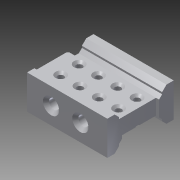
# Autodesk Inventor part: OnxyBelly
Saved by Autodesk Inventor 2015 (Build 190159000, 159)
## iProperties
Created: 2015-05-12
Part Number: OnxyBelly
Material: ABS Plastic
Document SubType Name: Modeling
Designer: Quinn
Density: 1.06 g/cm^3
Appearance: Smooth - White
Author: Quinn
Autodesk Inventor part; units mm, degrees
ref_plane "YZ Plane" through (0, 0, 0) normal (1, 0, 0) x (0, 1, 0)
ref_plane "XZ Plane" through (0, 0, 0) normal (0, 1, 0) x (-1, 0, 0)
ref_plane "XY Plane" through (0, 0, 0) normal (0, 0, 1) x (1, 0, 0)
sketch "Sketch1" plane through (0, 0, 0) normal (0, 1, 0) x (-1, 0, 0)
  line L0 (25, 21.5) -> (-25, 21.5)
  line L1 (-25, 21.5) -> (-25, -21.5)
  line L2 (-25, -21.5) -> (25, -21.5)
  line L3 (25, -21.5) -> (25, 21.5)
  line L4 (25, 21.5) -> (-25, 21.5)
  line L5 (-25, 21.5) -> (-25, 14)
  line L6 (-25, 14) -> (25, 14)
  line L7 (25, 14) -> (25, 21.5)
  line L8 (25, 0) -> (-25, 0)
  line L9 (-25, -14) -> (25, -14)
  line L10 (25, -14) -> (-25, -14)
  line L11 (-25, -14) -> (-25, -21.5)
  line L12 (-25, -21.5) -> (25, -21.5)
  line L13 (25, -21.5) -> (25, -14)
  point P0 (0, 0)
  point P1 (0, -21.5)
  dimension "d0" = 50
  dimension "d1" = 43
  dimension "d2" = 7.5
  constraints: 28 end point, 6 parallel, 3 horizontal, 3 midpoint, 3 perpendicular, 2 symmetric about line, 1 horizontal alignment, 1 point on line, 1 vertical alignment
  measures "d0" distance of L2.end L1.end
  measures "d1" distance of L1.end L0.end
  measures "d2" distance of L5.end L4.end
extrude "Extrusion1" add sketch "Sketch1" along normal blind 22 contours L3 L6 L1 L0 | L3 L2 L1 L9
ref_plane "Work Plane1" through (0, 11, 0) normal (0, 1, 0) x (1, 0, 0)
sketch "Sketch2" plane through (0, 11, 0) normal (0, 1, 0) x (1, 0, 0)
  line L0 (25, -14) -> (-25, -14) projected
  line L1 (25, -14) -> (-25, -14) projected
  line L2 (-25, 14) -> (25, 14) projected
  line L3 (-25, 14) -> (25, 14) projected
  line L4 (-25, -14) -> (25, -14)
  line L5 (25, -14) -> (25, 14)
  line L6 (25, 14) -> (-25, 14)
  line L7 (-25, 14) -> (-25, -14)
  point P0 (0, 0)
  constraints: 8 end point, 2 parallel, 1 horizontal, 1 perpendicular
extrude "Extrusion2" add sketch "Sketch2" along normal mid plane 10
chamfer "Chamfer1" distance 2 angle 45 4 edges at (0, 16, 14) (0, 16, -14) (0, 6, -14) (0, 6, 14)
sketch "Sketch3" plane through (0, 16, 0) normal (0, 1, 0) x (1, 0, 0)
  line L0 (-25, 12) -> (25, 12) projected
  line L1 (-25, 12) -> (-25, -12) projected
  line L2 (25, -12) -> (-25, -12) projected
  line L3 (25, -12) -> (25, 12) projected
  point P0 (0, 0)
sketch "Sketch4" plane through (0, 16, 0) normal (0, 1, 0) x (1, 0, 0)
  line L0 (25, 12) -> (-25, 12) projected
  line L1 (-25, 12) -> (25, 12) projected
  line L2 (-25, 12) -> (-25, -12) projected
  line L3 (25, -12) -> (-25, -12) projected
  line L4 (25, -12) -> (25, 12) projected
  line L5 (-25, 0) -> (25, 0)
  line L6 (-25, 0) -> (-25, -12)
  line L7 (-25, -6) -> (25, -6)
  line L8 (0, 0) -> (0, -12)
  line L9 (-25, 0) -> (-12.5, 0)
  line L10 (-12.5, 0) -> (-12.5, -12)
  line L11 (-18.75, 0) -> (-18.75, -12)
  circle A0 centre (-18.75, -6) radius 2
  circle A1 centre (-6.25, -6) radius 2
  circle A2 centre (6.25, -6) radius 2
  circle A3 centre (18.75, -6) radius 2
  circle A4 centre (-18.75, 6) radius 2
  circle A5 centre (-6.25, 6) radius 2
  circle A6 centre (6.25, 6) radius 2
  circle A7 centre (18.75, 6) radius 2
  dimension "d10" = 12.5
  dimension "d11" = 4
  dimension "d14" = 12.5
  constraints: 14 end point, 8 centre point, 6 midpoint, 4 point on line, 4 symmetric about line, 3 perpendicular, 1 collinear, 1 horizontal, 10 other
  measures "d10" distance of L5.start L9.end
  measures "d11" diameter of A0
  measures "d14" distance of A0.centre A1.centre
extrude "Extrusion3" cut sketch "Sketch4" against normal blind 27.4625 contours A3 L7 | L7 A3 | A0 L11 L7 | L7 L11 A0 | A0 L7 L11 | A1 L7 | L7 A1 | A2 L7 | L7 A2 | L7 A0 L11 | A4 | A5 | A6 | A7
chamfer "Chamfer2" distance 2.8 angle 45 4 edges at (0, 22, 14) (0, 22, -14) (0, 0, -14) (0, 0, 14)
sketch "Sketch5" plane through (-25, 0, 21.5) normal (-1, 0, 0) x (0, 0, 1)
  line L0 (-4.7, 0) -> (-7.5, 2.8) projected
  line L1 (-4.7, 0) -> (0, 0) projected
  line L2 (0, 0) -> (0, 22) projected
  line L3 (-4.7, 22) -> (0, 22) projected
  line L4 (-7.5, 19.2) -> (-4.7, 22) projected
  line L5 (-7.5, 18) -> (-7.5, 19.2) projected
  line L6 (-9.5, 16) -> (-7.5, 18) projected
  line L7 (-33.5, 16) -> (-9.5, 16) projected
  line L8 (-35.5, 18) -> (-33.5, 16) projected
  line L9 (-35.5, 18) -> (-35.5, 19.2) projected
  line L10 (-38.3, 22) -> (-35.5, 19.2) projected
  line L11 (-43, 22) -> (-38.3, 22) projected
  line L12 (-43, 0) -> (-43, 22) projected
  line L13 (-43, 0) -> (-38.3, 0) projected
  line L14 (-35.5, 2.8) -> (-38.3, 0) projected
  line L15 (-35.5, 2.8) -> (-35.5, 4) projected
  line L16 (-33.5, 6) -> (-35.5, 4) projected
  line L17 (-9.5, 6) -> (-33.5, 6) projected
  line L18 (-7.5, 4) -> (-9.5, 6) projected
  line L19 (-7.5, 2.8) -> (-7.5, 4) projected
  line L20 (-5.5, 3.6284) -> (-3.8716, 2)
  line L21 (-3.8716, 2) -> (-2, 2)
  line L22 (-2, 2) -> (-2, 20)
  line L23 (-2, 20) -> (-3.8716, 20)
  line L24 (-3.8716, 20) -> (-5.5, 18.3716)
  line L25 (-5.5, 18.3716) -> (-5.5, 17.1716)
  line L26 (-5.5, 17.1716) -> (-8.6716, 14)
  line L27 (-8.6716, 14) -> (-34.3284, 14)
  line L28 (-34.3284, 14) -> (-37.5, 17.1716)
  line L29 (-37.5, 17.1716) -> (-37.5, 18.3716)
  line L30 (-37.5, 18.3716) -> (-39.1284, 20)
  line L31 (-39.1284, 20) -> (-41, 20)
  line L32 (-41, 20) -> (-41, 2)
  line L33 (-41, 2) -> (-39.1284, 2)
  line L34 (-39.1284, 2) -> (-37.5, 3.6284)
  line L35 (-37.5, 3.6284) -> (-37.5, 4.8284)
  line L36 (-37.5, 4.8284) -> (-34.3284, 8)
  line L37 (-34.3284, 8) -> (-8.6716, 8)
  line L38 (-8.6716, 8) -> (-5.5, 4.8284)
  line L39 (-5.5, 4.8284) -> (-5.5, 3.6284)
  point P0 (-21.5, 0)
  dimension "d24" = 2
  constraints: 40 end point, 19 other
  measures "d24" distance between parallel lines of L0 L20
extrude "Extrusion4" cut sketch "Sketch5" against normal blind 2.5 contours L39 L38 L37 L36 L35 L34 L33 L32 L31 L30 L29 L28 L27 L26 L25 L24 L23 L22 L21 L20
sketch "Sketch6" plane through (-25, 0, 21.5) normal (0, 0, 1) x (1, 0, 0)
  line L0 (50, 16) -> (0, 16) projected
  line L1 (0, 6) -> (50, 6) projected
  line L2 (0, 0) -> (50, 0) projected
  line L3 (50, 0) -> (50, 22) projected
  line L4 (0, 22) -> (50, 22) projected
  line L5 (0, 0) -> (0, 22) projected
  line L6 (25, 0) -> (25, 22)
  line L7 (25, 11) -> (34.5, 11)
  line L8 (34.5, 11) -> (15.5, 11)
  circle A0 centre (34.5, 11) radius 3.25
  circle A1 centre (15.5, 11) radius 3.25
  dimension "d27" = 9.5
  dimension "d28" = 19
  dimension "d29" = 6.5
  dimension "d30" = 6.5
  constraints: 6 end point, 2 centre point, 2 coincident, 2 midpoint, 1 horizontal, 1 point on line
  measures "d27" distance of L7.start L7.end
  measures "d28" distance of L7.end L8.end
  measures "d29" diameter of A0
  measures "d30" diameter of A1
extrude "Extrusion5" cut sketch "Sketch6" against normal blind 6.5875 contours A0 | A1
mirror "Mirror1" about plane through (0, 0, 0) normal (0, 0, 1) of "Extrusion5"
chamfer "Chamfer3" distance 2 angle 45 4 edges at (-12.75, 11, -21.5) (6.25, 11, -21.5) (6.25, 11, 21.5) (-12.75, 11, 21.5)
chamfer "Chamfer4" distance 1.4 angle 45 16 edges at (-20.75, 6, 6) (-8.25, 6, 6) (4.25, 6, 6) (16.75, 6, 6) (16.75, 6, -6) (4.25, 6, -6) (-8.25, 6, -6) (-20.75, 6, -6) (-20.75, 16, -6) (-20.75, 16, 6) (-8.25, 16, 6) (-8.25, 16, -6) (4.25, 16, -6) (4.25, 16, 6) (16.75, 16, 6) (16.75, 16, -6)
sketch "Sketch7" plane through (25, 0, -21.5) normal (1, 0, 0) x (0, 0, -1)
  line L0 (-35.5, 2.8) -> (-38.3, 0) projected
  line L1 (-35.5, 2.8) -> (-35.5, 4) projected
  line L2 (-33.5, 6) -> (-35.5, 4) projected
  line L3 (-9.5, 6) -> (-33.5, 6) projected
  line L4 (-7.5, 4) -> (-9.5, 6) projected
  line L5 (-7.5, 2.8) -> (-7.5, 4) projected
  line L6 (-4.7, 0) -> (-7.5, 2.8) projected
  line L7 (-4.7, 0) -> (0, 0) projected
  line L8 (0, 0) -> (0, 22) projected
  line L9 (-4.7, 22) -> (0, 22) projected
  line L10 (-7.5, 19.2) -> (-4.7, 22) projected
  line L11 (-7.5, 18) -> (-7.5, 19.2) projected
  line L12 (-9.5, 16) -> (-7.5, 18) projected
  line L13 (-33.5, 16) -> (-9.5, 16) projected
  line L14 (-35.5, 18) -> (-33.5, 16) projected
  line L15 (-35.5, 18) -> (-35.5, 19.2) projected
  line L16 (-38.3, 22) -> (-35.5, 19.2) projected
  line L17 (-43, 22) -> (-38.3, 22) projected
  line L18 (-43, 0) -> (-43, 22) projected
  line L19 (-43, 0) -> (-38.3, 0) projected
  line L20 (-9.5, 6) -> (-33.5, 6)
  line L21 (-33.5, 6) -> (-33.5, 16)
  line L22 (-33.5, 16) -> (-9.5, 16)
  line L23 (-9.5, 16) -> (-9.5, 6)
  point P0 (-21.5, 0)
  constraints: 8 end point, 2 parallel, 1 horizontal, 1 perpendicular
extrude "Extrusion6" add sketch "Sketch7" along normal blind 2 contours L0 L19 L18 L17 L16 L15 L14 L21 L2 L1 | L23 L12 L11 L10 L9 L8 L7 L6 L5 L4
sketch "Sketch8" plane through (-22.5, 0, 21.5) normal (-1, 0, 0) x (0, 0, 1)
  line L0 (-3.8716, 2) -> (-5.5, 3.6284) projected
  line L1 (-2, 2) -> (-3.8716, 2) projected
  line L2 (-2, 20) -> (-2, 2) projected
  line L3 (-3.8716, 20) -> (-2, 20) projected
  line L4 (-5.5, 18.3716) -> (-3.8716, 20) projected
  line L5 (-5.5, 17.1716) -> (-5.5, 18.3716) projected
  line L6 (-8.6716, 14) -> (-5.5, 17.1716) projected
  line L7 (-34.3284, 14) -> (-8.6716, 14) projected
  line L8 (-37.5, 17.1716) -> (-34.3284, 14) projected
  line L9 (-37.5, 18.3716) -> (-37.5, 17.1716) projected
  line L10 (-39.1284, 20) -> (-37.5, 18.3716) projected
  line L11 (-41, 20) -> (-39.1284, 20) projected
  line L12 (-41, 2) -> (-41, 20) projected
  line L13 (-39.1284, 2) -> (-41, 2) projected
  line L14 (-37.5, 3.6284) -> (-39.1284, 2) projected
  line L15 (-37.5, 4.8284) -> (-37.5, 3.6284) projected
  line L16 (-34.3284, 8) -> (-37.5, 4.8284) projected
  line L17 (-8.6716, 8) -> (-34.3284, 8) projected
  line L18 (-5.5, 4.8284) -> (-8.6716, 8) projected
  line L19 (-5.5, 3.6284) -> (-5.5, 4.8284) projected
  line L20 (-8.6716, 8) -> (-8.6716, 14)
  line L21 (-2, 11) -> (-8.6716, 11)
  line L22 (-34.3284, 8) -> (-34.3284, 14)
  point P0 (-21.5, 0)
  constraints: 6 end point, 2 midpoint, 1 point on line, 1 vertical
ref_plane "Work Plane2" through (0, 11, 0) normal (0, -1, 0) x (1, 0, 0)
extrude "Extrusion7" add sketch "Sketch8" along normal blind 10 contours L17 L22 L7 L20
chamfer "Chamfer5" distance 1.4 angle 45 4 edges at (-28.75, 14, 12.8284) (-28.75, 14, -12.8284) (-28.75, 8, -12.8284) (-28.75, 8, 12.8284)
sketch "Sketch11" plane through (-32.5, 8, 11.4284) normal (0, -1, 0) x (1, 0, 0)
  line L0 (0, 0) -> (7.5, 0) projected
  line L1 (0, -22.8569) -> (0, 0) projected
  line L2 (7.5, -22.8569) -> (0, -22.8569) projected
  line L3 (7.5, 0) -> (7.5, -22.8569) projected
  line L4 (0, -22.8569) -> (3, -22.8569)
  line L5 (3, -22.8569) -> (3, 0)
  line L6 (3, 0) -> (0, 0)
  line L7 (0, 0) -> (0, -22.8569)
  line L8 (3, -11.4284) -> (0, -11.4284)
  line L9 (3, 0) -> (3, -5.714)
  line L10 (3, -5.714) -> (0, -5.714)
  line L11 (3, -2.857) -> (0, -2.857)
  line L12 (3, -5.714) -> (3, -8.571)
  point P0 (32.5, -11.4284)
  dimension "d46" = 3
  dimension "d47" = 5.714
  dimension "d48" = 2.857
  constraints: 18 end point, 5 point on line, 3 midpoint, 3 perpendicular, 2 parallel, 1 horizontal
  measures "d46" distance of L6.end L5.end
  measures "d47" distance of L5.end L9.end
  measures "d48" distance of L9.end L12.end
extrude "Extrusion8" add sketch "Sketch11" along normal blind 8 contours L0 L5 L11 L1 | L11 L5 L10 L1 | L10 L5 L8 L1 | L8 L5 L2 L1
sketch "Sketch12" plane through (-32.5, 0, 21.5) normal (-1, 0, 0) x (0, 0, 1)
  line L0 (-8.6716, 9.4) -> (-10.0716, 8) projected
  line L1 (-8.6716, 9.4) -> (-8.6716, 12.6) projected
  line L2 (-10.0716, 14) -> (-8.6716, 12.6) projected
  line L3 (-10.0716, 14) -> (-32.9284, 14) projected
  line L4 (-34.3284, 12.6) -> (-32.9284, 14) projected
  line L5 (-34.3284, 12.6) -> (-34.3284, 9.4) projected
  line L6 (-32.9284, 8) -> (-34.3284, 9.4) projected
  line L7 (-32.9284, 8) -> (-32.9284, 0) projected
  line L8 (-10.0716, 0) -> (-32.9284, 0) projected
  line L9 (-10.0716, 8) -> (-10.0716, 0) projected
  line L10 (-10.0716, 4) -> (-32.9284, 4)
  circle A0 centre (-14.0716, 4) radius 2.5
  circle A1 centre (-21.5, 4) radius 2.5
  circle A2 centre (-28.9284, 4) radius 2.5
  point P0 (-21.5, 0)
  dimension "d51" = 5
  dimension "d52" = 5
  dimension "d53" = 5
  constraints: 3 centre point, 3 midpoint, 2 end point, 2 point on line
  measures "d51" diameter of A0
  measures "d52" diameter of A1
  measures "d53" diameter of A2
extrude "Extrusion9" cut sketch "Sketch12" against normal blind 5 contours A0 L10 | L10 A0 | A2 L10 | L10 A2
extrude "Extrusion10" cut sketch "Sketch12" against normal through all contours A1 L10 | L10 A1
chamfer "Chamfer6" distance 1 angle 45 7 edges at (-29.5, 0, 0) (-32.5, 0, 0) (-31, 0, 11.4284) (-31, 0, -11.4284) (-32.5, 14, 0) (-32.5, 11, 12.8284) (-32.5, 11, -12.8284)
sketch "Sketch13" plane through (-29.5, 8, 11.4284) normal (1, 0, 0) x (0, 0, -1)
  line L0 (22.8569, -7) -> (0, -7) projected
  line L1 (22.8569, 0) -> (22.8569, -7) projected
  line L2 (0, 0) -> (22.8569, 0) projected
  line L3 (0, 0) -> (0, -7) projected
  circle A0 centre (11.4284, -4) radius 2.5 projected
  circle A1 centre (18.8569, -4) radius 2.5 projected
  circle A2 centre (4, -4) radius 2.5 projected
  line L4 (16.3569, -4) -> (13.9284, -4)
  line L5 (15.1426, -4) -> (15.1426, 0)
  line L6 (8.9284, -4) -> (6.5, -4)
  line L7 (7.7142, -4) -> (7.7142, 0)
  line L8 (8.4642, 0) -> (6.9642, 0)
  line L9 (6.9642, 0) -> (6.9642, -4)
  line L10 (6.9642, -4) -> (8.4642, -4)
  line L11 (8.4642, -4) -> (8.4642, 0)
  line L12 (8.4642, 0) -> (6.9642, -4) construction
  line L13 (6.9642, 0) -> (8.4642, -4) construction
  line L14 (15.8926, 0) -> (14.3926, 0)
  line L15 (14.3926, 0) -> (14.3926, -4)
  line L16 (14.3926, -4) -> (15.8926, -4)
  line L17 (15.8926, -4) -> (15.8926, 0)
  line L18 (15.8926, 0) -> (14.3926, -4) construction
  line L19 (14.3926, 0) -> (15.8926, -4) construction
  point P0 (11.4284, -8)
  point P1 (7.7142, -2)
  point P2 (15.1426, -2)
  dimension "d61" = 1.5
  dimension "d62" = 1.5
  constraints: 32 end point, 8 midpoint, 5 parallel, 5 point on line, 4 perpendicular, 2 horizontal, 2 horizontal alignment, 2 point on circle, 2 other
  measures "d61" distance of L10.end L9.end
  measures "d62" distance of L16.end L15.end
extrude "Extrusion11" add sketch "Sketch13" along normal blind 4 contours L17 L4 L5 L2 | L2 L7 L6 L9 | L5 L4 L15 L2 | L2 L11 L6 L7
chamfer "Chamfer7" distance 4 angle 45 2 edges at (-25.5, 4, -3.7142) (-25.5, 4, 3.7142)
offset faces "Size1" outward 7.938 faces at (-32.5, 10.8273, 0.1004)
offset faces "Size2" outward -1.588 faces at (-33.8183, 9.2466, -10.5102) (-33.8183, 9.2466, 10.5102)
body "Solid1"
